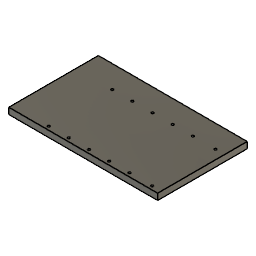
screw on plate (Autodesk Fusion 360 design; units mm, degrees)
Autodesk Fusion 360 part; units mm, degrees
sketch "Skizze1" plane through (0, 0, 0) normal (0, 0, 1) x (1, 0, 0)
  line L0 (0, 0) -> (-211, 0)
  line L1 (-211, 0) -> (-211, 127)
  line L2 (-211, 127) -> (0, 127)
  line L3 (0, 127) -> (0, 0)
  circle A0 centre (-13, 5) radius 1.625
  circle A1 centre (-13, 95) radius 1.625
  circle A2 centre (-45, 5) radius 1.625
  circle A3 centre (-45, 95) radius 1.625
  circle A4 centre (-73.6, 5) radius 1.625
  circle A5 centre (-73.6, 5) radius 1.625
  circle A6 centre (-102.2, 5) radius 1.625
  circle A7 centre (-130.8, 5) radius 1.625
  circle A8 centre (-159.4, 5) radius 1.625
  circle A9 centre (-73.6, 95) radius 1.625
  circle A10 centre (-102.2, 95) radius 1.625
  circle A11 centre (-159.4, 95) radius 1.625
  circle A12 centre (-130.8, 95) radius 1.625
  dimension "d1" = 211
  dimension "d2" = 127
  dimension "d3" = 3.25
  dimension "d4" = 13
  dimension "d5" = 5
  dimension "d6" = 3.25
  dimension "d7" = 13
  dimension "d8" = 90
  dimension "d9" = 3.25
  dimension "d10" = 32
  dimension "d11" = 3.25
  dimension "d12" = 3.25
  dimension "d13" = 28.6
  dimension "d14" = 3.25
  dimension "d15" = 3.25
  dimension "d16" = 3.25
  dimension "d17" = 3.25
  dimension "d18" = 3.25
  dimension "d19" = 3.25
  dimension "d20" = 3.25
  dimension "d21" = 3.25
  constraint horizontal L0
  constraint vertical L1
  constraint horizontal L2
  constraint vertical L3
  constraint coincident L0.start L3.end
  measures "d1" distance of L0.start L0.end
  measures "d2" distance of L0.start L2.end
  measures "d3" diameter of A0
  measures "d4" distance of L3 A0.centre
  measures "d5" distance of L0 A0.centre
  measures "d6" diameter of A1
  measures "d7" distance of L3 A1.centre
  measures "d8" distance of A0.centre A1.centre
  measures "d9" diameter of A2
  measures "d10" distance of A0.centre A2.centre
  measures "d11" diameter of A3
  measures "d12" diameter of A4
  measures "d13" distance of A2.centre A4.centre
  measures "d14" diameter of A5
  measures "d15" diameter of A6
  measures "d16" diameter of A7
  measures "d17" diameter of A8
  measures "d18" diameter of A9
  measures "d19" diameter of A10
  measures "d20" diameter of A12
  measures "d21" diameter of A11
extrude "Extrusion1" add sketch "Skizze1" along normal blind 9
